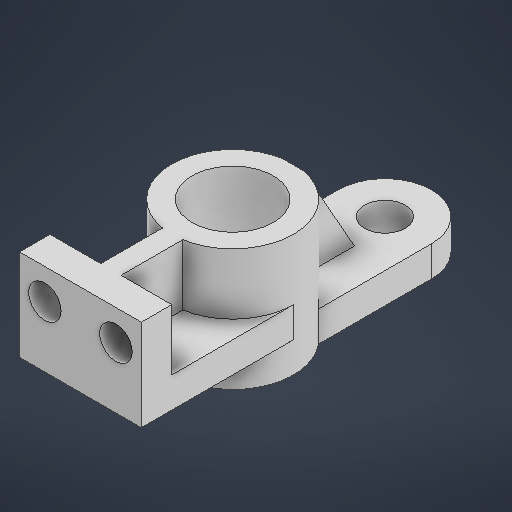
# Autodesk Inventor part: Pieza3
Saved by Autodesk Inventor 2026 (Build 300175000, 175)
## iProperties
Created: 2025-04-04
Part Number: Pieza3
Material: Genérico
Document SubType Name: Modeling
Designer: LabB305
Density: 1 g/cm^3
Appearance: Valor por defecto
Author: LabB305
Autodesk Inventor part; units mm, degrees
ref_plane "YZ Plane" through (0, 0, 0) normal (1, 0, 0) x (0, 1, 0)
ref_plane "XZ Plane" through (0, 0, 0) normal (0, 1, 0) x (-1, 0, 0)
ref_plane "XY Plane" through (0, 0, 0) normal (0, 0, 1) x (1, 0, 0)
sketch "Boceto1" plane through (0, 0, 0) normal (0, 1, 0) x (-1, 0, 0)
  circle A0 centre (0, 0) radius 20
  circle A1 centre (0, 0) radius 30
  line L0 (0, 0) -> (0, 60)
  line L1 (0, 60) -> (5, 60)
  line L2 (5, 60) -> (-5, 60)
  line L3 (-5, 60) -> (-5, 0)
  line L4 (-5, 0) -> (5, 0)
  line L5 (5, 0) -> (5, 60)
  line L6 (0, 60) -> (30, 60)
  line L7 (30, 60) -> (-30, 60)
  line L8 (-30, 60) -> (-30, 75)
  line L9 (-30, 75) -> (30, 75)
  line L10 (30, 75) -> (30, 60)
  point P0 (-5, 29.5804)
  point P1 (5, 29.5804)
  dimension "d0" = 40
  dimension "d1" = 60
  dimension "d2" = 60
  dimension "d3" = 5
  dimension "d4" = 10
  dimension "d5" = 30
  dimension "d6" = 60
  dimension "d7" = 15
  constraints: 22 end point, 4 parallel, 3 horizontal, 3 perpendicular, 2 centre point, 2 coincident, 1 vertical
  measures "d0" diameter of A0
  measures "d1" diameter of A1
  measures "d2" distance of L0.start L0.end
  measures "d3" distance of L0.end L1.end
  measures "d4" distance of L4.end L3.end
  measures "d5" distance of L0.end L6.end
  measures "d6" distance of L8.end L9.end
  measures "d7" distance of L7.end L8.end
extrude "Extrusión1" add sketch "Boceto1" along normal blind 60
sketch "Boceto2" plane through (30, 0, 75) normal (1, 0, 0) x (0, 0, -1)
  line L0 (0, 60) -> (15, 60) projected
  line L1 (0, 60) -> (0, 15)
  line L2 (0, 0) -> (0, 60) projected
  line L3 (0, 15) -> (75, 15)
  line L4 (75, 15) -> (75, 30)
  line L5 (75, 30) -> (15, 30)
  line L6 (15, 0) -> (15, 60) projected
  point P0 (75, 0)
  point P1 (15, 15)
  dimension "d10" = 45
  dimension "d11" = 15
  constraints: 8 end point, 1 horizontal, 1 midpoint, 1 perpendicular, 1 point on line
  measures "d10" distance of L0.start L1.end
  measures "d11" distance of L3.end L4.end
extrude "Extrusión2" add sketch "Boceto2" against normal blind 60 contours L5 L4 L3 L6
sketch "Boceto3" plane through (30, 0, 75) normal (1, 0, 0) x (0, 0, -1)
  line L0 (45.4196, 15) -> (15, 15) projected
  line L1 (15, 15) -> (0, 15)
  line L2 (0, 0) -> (0, 60) projected
  line L3 (45.4196, 0) -> (15, 0) projected
  line L4 (0, 15) -> (45.4196, 15)
  line L5 (45.4196, 15) -> (45.4196, 0)
  line L6 (45.4196, 0) -> (0, 0)
  line L7 (0, 0) -> (0, 15)
  point P0 (75, 0)
  constraints: 10 end point, 2 horizontal, 2 parallel, 1 perpendicular, 1 point on line
extrude "Extrusión3" cut sketch "Boceto3" against normal blind 60
sketch "Boceto4" plane through (-30, 60, 75) normal (0, 0, 1) x (1, 0, 0)
  line L0 (60, 0) -> (0, 0) projected
  line L1 (30, 0) -> (47.5, 0)
  line L2 (47.5, 0) -> (47.5, -15)
  line L3 (30, 0) -> (30, -5.3607)
  circle A0 centre (47.5, -15) radius 8
  circle A1 centre (12.5, -15) radius 8
  point P0 (30, -60)
  point P1 (35, 0)
  point P2 (25, 0)
  dimension "d16" = 17.5
  dimension "d17" = 15
  dimension "d18" = 16
  constraints: 6 end point, 2 centre point, 2 vertical, 1 coincident, 1 midpoint, 1 point on line, 1 symmetric about line, 1 other
  measures "d16" distance of L1.start L1.end
  measures "d17" distance of L1.end L2.end
  measures "d18" diameter of A0
extrude "Extrusión4" cut sketch "Boceto4" against normal blind 15
sketch "Boceto5" plane through (0, 60, 0) normal (0, 1, 0) x (1, 0, 0)
  circle A0 centre (0, 0) radius 20
  dimension "d21" = 40
  constraints: 1 centre point, 1 coincident
  measures "d21" diameter of A0
extrude "Extrusión5" cut sketch "Boceto5" against normal blind 60
sketch "Boceto6" plane through (0, 0, 0) normal (0, -1, 0) x (1, 0, 0)
  line L0 (0, 0) -> (0, -75)
  circle A0 centre (0, -75) radius 10
  circle A1 centre (0, -75) radius 23
  line L1 (0, -75) -> (23, -75)
  arc A2 (-5, 29.5804) -> (5, 29.5804) centre (0, 0) ccw projected
  line L2 (23, -19.2614) -> (23, -75)
  line L3 (-23, -19.2614) -> (-23, -75)
  dimension "d24" = 75
  dimension "d25" = 20
  dimension "d26" = 46
  constraints: 8 end point, 5 point on circle, 2 centre point, 2 coincident, 2 vertical, 1 horizontal, 1 tangent
  measures "d24" distance of L0.start L0.end
  measures "d25" diameter of A0
  measures "d26" diameter of A1
extrude "Extrusión6" add sketch "Boceto6" against normal blind 15 contours A2 L2 A1 L0 | L0 A1 L3 A2 | A1 L1 A0 L0 | L0 A0 L1 A1
sketch "Boceto7" plane through (0, 60, 0) normal (0, 1, 0) x (1, 0, 0)
  arc A0 (5, -29.5804) -> (-5, -29.5804) centre (0, 0) ccw projected
  line L0 (0, 30) -> (0, 55)
  line L1 (0, 55) -> (5, 55)
  line L2 (5, 29.5804) -> (5, 55)
  line L3 (0, 55) -> (-5, 55)
  line L4 (-5, 29.5804) -> (-5, 55)
  arc A1 (5, 29.5804) -> (-5, 29.5804) centre (0, 0) ccw
  dimension "d29" = 25
  dimension "d30" = 5
  constraints: 10 end point, 6 point on circle, 2 symmetric about line, 2 vertical, 1 centre point, 1 perpendicular
  measures "d29" distance of L0.start L0.end
  measures "d30" distance of L0.end L1.end
extrude "Extrusión7" add sketch "Boceto7" against normal blind 45
sketch "Boceto8" plane through (-5, 60, -55) normal (-1, 0, 0) x (0, 0, 1)
  line L0 (0, 0) -> (0, -45) projected
  line L1 (84.5804, 0) -> (25.4196, 0) projected
  line L2 (0, -45) -> (25.4196, 0)
  line L3 (35.7386, -45) -> (25.4196, -45) projected
  line L4 (25.4196, 0) -> (25.4196, -45)
  line L5 (25.4196, -45) -> (0, -45)
  line L6 (0, -45) -> (0, 0)
  line L7 (25.4196, 0) -> (0, 0)
  point P0 (55, -60)
  constraints: 10 end point, 3 perpendicular, 1 collinear, 1 point on line
extrude "Extrusión8" cut sketch "Boceto8" against normal blind 45 contours L7 L2 L0
